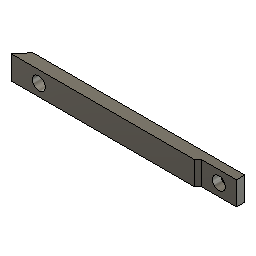
Buzzer Clamp v7 (Autodesk Fusion 360 design; units mm, degrees)
Autodesk Fusion 360 part; units mm, degrees
sketch "Sketch1" plane through (0, 0, 0) normal (0, 0, 1) x (1, 0, 0)
  line L0 (0, 0) -> (45.72, 0)
  line L1 (45.72, 0) -> (45.72, 5.08)
  line L2 (45.72, 5.08) -> (0, 5.08)
  line L3 (0, 5.08) -> (0, 0)
  circle A0 centre (3.81, 2.54) radius 1.397
  circle A1 centre (41.91, 2.54) radius 1.397
  dimension "d1" = 45.72
  dimension "d2" = 5.08
  dimension "d3" = 2.794
  dimension "d4" = 2.54
  dimension "d5" = 3.81
  dimension "d6" = 2.794
  dimension "d7" = 2.54
  dimension "d8" = 3.81
  constraint horizontal L0
  constraint vertical L1
  constraint horizontal L2
  constraint vertical L3
  constraint coincident L0.start L3.end
  measures "d1" distance of L0.start L0.end
  measures "d2" distance of L0.start L2.end
  measures "d3" diameter of A0
  measures "d4" distance of L2 A0.centre
  measures "d5" distance of L3 A0.centre
  measures "d6" diameter of A1
  measures "d7" distance of L2 A1.centre
  measures "d8" distance of L1 A1.centre
extrude "Extrude1" add sketch "Sketch1" along normal blind 2.54
draft "Draft1" angle 40 neutral plane through (0, 0, 0) pull (0, 0, -1) 1 faces at (0, 3.3867, 0.8467)
sketch "Sketch3" plane through (0, 0, 2.54) normal (0, 0, 1) x (1, 0, 0)
  circle A0 centre (3.81, 2.54) radius 1.397
  circle A1 centre (41.91, 2.54) radius 1.397
  line L0 (-2.1313, 5.08) -> (-2.1313, 0)
  line L1 (-2.1313, 0) -> (45.72, 0)
  line L2 (45.72, 0) -> (45.72, 5.08)
  line L3 (45.72, 5.08) -> (-2.1313, 5.08)
  line L4 (45.72, 5.08) -> (38.1, 5.08)
  line L5 (38.1, 5.08) -> (38.1, 0)
  line L6 (38.1, 0) -> (45.72, 0)
  line L7 (45.72, 0) -> (45.72, 5.08)
  dimension "d16" = 7.62
  dimension "d17" = 5.08
  constraint horizontal L4
  constraint vertical L5
  constraint horizontal L6
  constraint vertical L7
  constraint coincident L2.end L3.start
  measures "d16" distance of L2.end L4.end
  measures "d17" distance of L2.end L1.end
extrude "Extrude3" cut sketch "Sketch3" against normal blind 0.762 contours L1 L2 L3 L4 L5 L6 L7
chamfer "Chamfer1" distance 0.762 angle 45 1 edges at (38.1, 2.54, 2.54)
